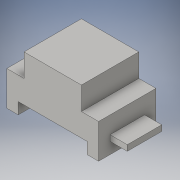
# Autodesk Inventor part: Part 1
Saved by Autodesk Inventor 2016 (Build 200138000, 138)
## iProperties
Created: 2016-10-21
Part Number: Part 1
Material: Generic
Document SubType Name: Modeling
Designer: 196918
Density: 1 g/cm^3
Appearance: Default
Author: 196918
Autodesk Inventor part; units mm, degrees
ref_plane "YZ Plane" through (0, 0, 0) normal (1, 0, 0) x (0, 1, 0)
ref_plane "XZ Plane" through (0, 0, 0) normal (0, 1, 0) x (-1, 0, 0)
ref_plane "XY Plane" through (0, 0, 0) normal (0, 0, 1) x (1, 0, 0)
sketch "Sketch1" plane through (0, 0, 0) normal (1, 0, 0) x (0, 1, 0)
  line L0 (9.5985, 34.7638) -> (-15.8015, 34.7638)
  line L1 (-15.8015, 34.7638) -> (-15.8015, -28.7362)
  line L2 (-15.8015, -28.7362) -> (9.5985, -28.7362)
  line L3 (9.5985, -28.7362) -> (9.5985, 34.7638)
  point P0 (0, 0)
  dimension "d0" = 25.4
  dimension "d1" = 63.5
  constraints: 8 end point, 2 parallel, 1 horizontal, 1 perpendicular
  measures "d0" distance of L2.end L1.end
  measures "d1" distance of L1.end L0.end
extrude "Extrusion1" add sketch "Sketch1" along normal blind 63.5
sketch "Sketch2" plane through (0, -15.8015, 34.7638) normal (0, 0, 1) x (1, 0, 0)
  line L0 (0, 0) -> (63.5, 0) projected
  line L1 (31.75, 0) -> (-19.05, 0)
  line L2 (-19.05, 0) -> (82.55, 0)
  line L3 (82.55, 0) -> (82.55, -25.4)
  line L4 (82.55, -25.4) -> (-19.05, -25.4)
  line L5 (-19.05, -25.4) -> (-19.05, 0)
  point P0 (0, 15.8015)
  dimension "d4" = 50.8
  dimension "d5" = 101.6
  dimension "d6" = 25.4
  constraints: 10 end point, 3 perpendicular, 1 collinear, 1 midpoint, 1 point on line
  measures "d4" distance of L1.start L1.end
  measures "d5" distance of L1.end L2.end
  measures "d6" distance of L2.end L3.end
extrude "Extrusion2" add sketch "Sketch2" against normal blind 63.5
sketch "Sketch3" plane through (0, 9.5985, 34.7638) normal (0, 0, 1) x (1, 0, 0)
  line L0 (82.55, -50.8) -> (-19.05, -50.8) projected
  line L1 (-19.05, -50.8) -> (-19.05, -63.5)
  line L2 (-19.05, -63.5) -> (-6.35, -63.5)
  line L3 (-6.35, -63.5) -> (-6.35, -50.8)
  line L4 (82.55, -50.8) -> (82.55, -63.5)
  line L5 (82.55, -63.5) -> (69.85, -63.5)
  line L6 (69.85, -63.5) -> (69.85, -50.8)
  point P0 (0, -9.5985)
  dimension "d9" = 12.7
  dimension "d10" = 12.7
  dimension "d11" = 12.7
  dimension "d12" = 12.7
  constraints: 12 end point, 4 point on line, 3 perpendicular, 1 vertical
  measures "d9" distance of L0.end L1.end
  measures "d10" distance of L1.end L2.end
  measures "d11" distance of L0.start L4.end
  measures "d12" distance of L4.end L5.end
extrude "Extrusion3" add sketch "Sketch3" against normal blind 63.5
sketch "Sketch4" plane through (82.55, -15.8015, 34.7638) normal (1, 0, 0) x (0, 0, -1)
  line L0 (0, 0) -> (63.5, 0) projected
  line L1 (31.75, -19.05) -> (12.7, -19.05)
  line L2 (12.7, -19.05) -> (50.8, -19.05)
  line L3 (50.8, -19.05) -> (50.8, -25.4)
  line L4 (0, -25.4) -> (63.5, -25.4) projected
  line L5 (50.8, -25.4) -> (12.7, -25.4)
  line L6 (12.7, -25.4) -> (12.7, -19.05)
  point P0 (34.7638, 15.8015)
  dimension "d16" = 19.05
  dimension "d17" = 38.1
  dimension "d18" = 6.35
  dimension "d19" = 38.1
  dimension "d20" = 6.35
  constraints: 10 end point, 3 point on line
  measures "d16" distance of L1.start L1.end
  measures "d17" distance of L1.end L2.end
  measures "d18" distance of L2.end L3.end
  measures "d19" distance of L3.end L5.end
  measures "d20" distance of L5.end L1.end
extrude "Extrusion4" add sketch "Sketch4" along normal blind 19.05
body "Solid1"
